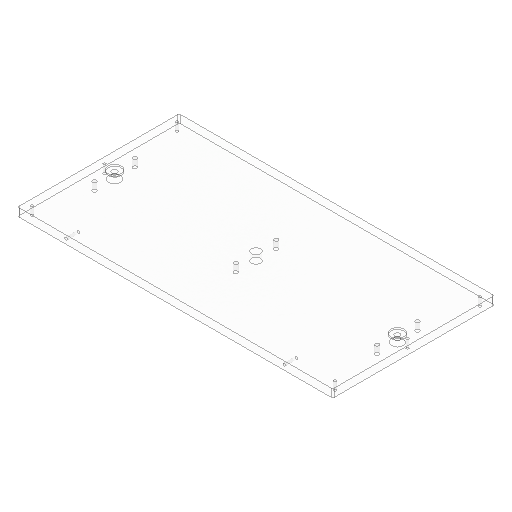
# Autodesk Inventor part: DLT-01-231B
Saved by Autodesk Inventor 2025.2 (Build 292293000, 293)
## iProperties
Company: Delta
Created: 2024-10-16
Part Number: DLT-01-231B
Material: Acrílico TP
Document SubType Name: Modeling
Designer: Willian Pinheiro
Density: 1.19 g/cm^3
Appearance: Transparent - Clear
Project: DLT
Description: Base Pressor B
Mass: 923.478 g
Surface Area: 1693.15 cm^2
Volume: 776.032 cm^3
Acabamento: N/A
Dimensões: 10 x 200 x 390 mm
Total: 1
Author: Willian Pinheiro
Revision Number: 00
Autodesk Inventor part; units mm, degrees
ref_plane "YZ Plane" through (0, 0, 0) normal (1, 0, 0) x (0, 1, 0)
ref_plane "XZ Plane" through (0, 0, 0) normal (0, 1, 0) x (-1, 0, 0)
ref_plane "XY Plane" through (0, 0, 0) normal (0, 0, 1) x (1, 0, 0)
sketch "Sketch1" plane through (0, 0, 0) normal (0, 0, 1) x (1, 0, 0)
  line L0 (0, -252.5291) -> (0, 252.5291) construction
  line L1 (-273, 0) -> (273, 0) construction
  line L2 (-195, 100) -> (195, 100)
  line L3 (195, 100) -> (195, -100)
  line L4 (195, -100) -> (-195, -100)
  line L5 (-195, -100) -> (-195, 100)
  line L6 (-178.1654, -28.1654) -> (-178.1654, 28.1654) construction
  line L7 (-178.1654, 28.1654) -> (178.1654, 28.1654) construction
  line L8 (178.1654, 28.1654) -> (178.1654, -28.1654) construction
  line L9 (178.1654, -28.1654) -> (-178.1654, -28.1654) construction
  circle A0 centre (0, 0) radius 180.3779 construction
  line L10 (-175, 25) -> (-175, -25) construction
  line L11 (-175, -25) -> (175, -25) construction
  line L12 (175, -25) -> (175, 25) construction
  line L13 (175, 25) -> (-175, 25) construction
  circle A1 centre (-175, 0) radius 6 construction
  point P0 (175, 0)
  point P1 (0, 25)
  point P2 (0, -25)
  dimension "d0" = 390
  dimension "d1" = 200
  dimension "d5" = 350
  dimension "d6" = 360.7559
  dimension "d14" = 350
  dimension "d15" = 12
  dimension "d54" = 353.5534
  dimension "d104" = 350
  dimension "d105" = 50
  constraints: 24 end point, 7 parallel, 6 coincident, 3 perpendicular, 3 point on circle, 2 centre point, 2 midpoint, 1 horizontal, 1 point on line, 1 symmetric about line, 5 other
  measures "d0" distance of L2.start L2.end
  measures "d1" distance between parallel lines of L4 L2
  measures "d5" distance between parallel lines of L12 L10
  measures "d6" diameter of A0
  measures "d14" distance of point (175, 0) point (-175, 0)
  measures "d15" diameter of A1
  measures "d54" distance of point (175, 25) point (-175, -25)
  measures "d104" distance of L12.end L10.start
  measures "d105" distance of L10.start L10.end
extrude "Extrusion1" add sketch "Sketch1" along normal blind 10
sketch "Sketch2" plane through (0, 0, 10) normal (0, 0, 1) x (1, 0, 0)
  point P0 (0, 0)
  point P1 (-175, -25)
  point P2 (-175, 25)
  point P3 (175, 25)
  point P4 (175, -25)
  point P5 (-175, 0)
  point P6 (175, 0)
  point P7 (0, 25)
  point P8 (0, -25)
hole "Hole1" at (-175, -25, 10) at (175, 25, 10) at (-175, 25, 10) at (175, -25, 10) at (0, 25, 10) at (0, -25, 10) direction (0, 0, -1) diameter 4.917 end through all thread size "M6x1" class "6H" standard "ISO Metric profile"
hole "Hole2" at (-175, 0, 10) at (175, 0, 10) direction (0, 0, -1) diameter 6.5 end through all counterbore diameter 16.5 counterbore depth 2
sketch "Sketch3" plane through (0, 0, 10) normal (0, 0, 1) x (1, 0, 0)
  line L0 (195, 100) -> (-195, 100) construction
  line L1 (-195, -100) -> (195, -100) construction
  line L2 (-195, 100) -> (-195, -100) construction
  line L3 (-273, 0) -> (273, 0) construction
  line L4 (0, -140) -> (0, 140) construction
  line L5 (195, -100) -> (195, 100) construction
  line L6 (-180, 90) -> (180, 90) construction
  line L7 (180, 90) -> (180, -90) construction
  line L8 (180, -90) -> (-180, -90) construction
  line L9 (-180, -90) -> (-180, 90) construction
  point P0 (0, 0)
  point P1 (-170, 80)
  point P2 (-150, 80)
  point P3 (-150, 80)
  point P4 (-130, 80)
  point P5 (-110, 80)
  point P6 (-90, 80)
  point P7 (-70, 80)
  point P8 (-50, 80)
  point P9 (-30, 80)
  point P10 (-10, 80)
  point P11 (10, 80)
  point P12 (30, 80)
  point P13 (50, 80)
  point P14 (70, 80)
  point P15 (90, 80)
  point P16 (110, 80)
  point P17 (130, 80)
  point P18 (150, 80)
  point P19 (170, 80)
  point P20 (-170, 60)
  point P21 (-150, 60)
  point P22 (-130, 60)
  point P23 (-110, 60)
  point P24 (-90, 60)
  point P25 (-70, 60)
  point P26 (-50, 60)
  point P27 (-30, 60)
  point P28 (-10, 60)
  point P29 (10, 60)
  point P30 (30, 60)
  point P31 (50, 60)
  point P32 (70, 60)
  point P33 (90, 60)
  point P34 (110, 60)
  point P35 (130, 60)
  point P36 (150, 60)
  point P37 (170, 60)
  point P38 (-170, 40)
  point P39 (-150, 40)
  point P40 (-130, 40)
  point P41 (-110, 40)
  point P42 (-90, 40)
  point P43 (-70, 40)
  point P44 (-50, 40)
  point P45 (-30, 40)
  point P46 (-10, 40)
  point P47 (10, 40)
  point P48 (30, 40)
  point P49 (50, 40)
  point P50 (70, 40)
  point P51 (90, 40)
  point P52 (110, 40)
  point P53 (130, 40)
  point P54 (150, 40)
  point P55 (170, 40)
  point P56 (-170, 20)
  point P57 (-150, 20)
  point P58 (-130, 20)
  point P59 (-110, 20)
  point P60 (-90, 20)
  point P61 (-70, 20)
  point P62 (-50, 20)
  point P63 (-30, 20)
  point P64 (-10, 20)
  point P65 (10, 20)
  point P66 (30, 20)
  point P67 (50, 20)
  point P68 (70, 20)
  point P69 (90, 20)
  point P70 (110, 20)
  point P71 (130, 20)
  point P72 (150, 20)
  point P73 (170, 20)
  point P74 (-170, 0)
  point P75 (-150, 0)
  point P76 (-130, 0)
  point P77 (-110, 0)
  point P78 (-90, 0)
  point P79 (-70, 0)
  point P80 (-50, 0)
  point P81 (-30, 0)
  point P82 (-10, 0)
  point P83 (10, 0)
  point P84 (30, 0)
  point P85 (50, 0)
  point P86 (70, 0)
  point P87 (90, 0)
  point P88 (110, 0)
  point P89 (130, 0)
  point P90 (150, 0)
  point P91 (170, 0)
  point P92 (-170, -20)
  point P93 (-150, -20)
  point P94 (-130, -20)
  point P95 (-110, -20)
  point P96 (-90, -20)
  point P97 (-70, -20)
  point P98 (-50, -20)
  point P99 (-30, -20)
  point P100 (-10, -20)
  point P101 (10, -20)
  point P102 (30, -20)
  point P103 (50, -20)
  point P104 (70, -20)
  point P105 (90, -20)
  point P106 (110, -20)
  point P107 (130, -20)
  point P108 (150, -20)
  point P109 (170, -20)
  point P110 (-170, -40)
  point P111 (-150, -40)
  point P112 (-130, -40)
  point P113 (-110, -40)
  point P114 (-90, -40)
  point P115 (-70, -40)
  point P116 (-50, -40)
  point P117 (-30, -40)
  point P118 (-10, -40)
  point P119 (10, -40)
  point P120 (30, -40)
  point P121 (50, -40)
  point P122 (70, -40)
  point P123 (90, -40)
  point P124 (110, -40)
  point P125 (130, -40)
  point P126 (150, -40)
  point P127 (170, -40)
  point P128 (-170, -60)
  point P129 (-150, -60)
  point P130 (-130, -60)
  point P131 (-110, -60)
  point P132 (-90, -60)
  point P133 (-70, -60)
  point P134 (-50, -60)
  point P135 (-30, -60)
  point P136 (-10, -60)
  point P137 (10, -60)
  point P138 (30, -60)
  point P139 (50, -60)
  point P140 (70, -60)
  point P141 (90, -60)
  point P142 (110, -60)
  point P143 (130, -60)
  point P144 (150, -60)
  point P145 (170, -60)
  point P146 (-170, -80)
  point P147 (-150, -80)
  point P148 (-130, -80)
  point P149 (-110, -80)
  point P150 (-90, -80)
  point P151 (-70, -80)
  point P152 (-50, -80)
  point P153 (-30, -80)
  point P154 (-10, -80)
  point P155 (10, -80)
  point P156 (30, -80)
  point P157 (50, -80)
  point P158 (70, -80)
  point P159 (90, -80)
  point P160 (110, -80)
  point P161 (130, -80)
  point P162 (150, -80)
  point P163 (170, -80)
  dimension "d25" = 10
  dimension "d26" = 360
  dimension "d27" = 180
  dimension "d28" = 10
  dimension "d29" = 10
  dimension "d30" = 20
  dimension "d33" = 20
  dimension "d36" = 20
  dimension "d39" = 15
  constraints: 8 end point, 1 horizontal, 1 horizontal alignment, 1 vertical, 163 other
  measures "d25" distance between parallel lines of L0 L6
  measures "d26" distance between parallel lines of L7 L9
  measures "d27" distance between parallel lines of L8 L6
  measures "d28" distance from line of point (-170, 80) L9
  measures "d29" distance from line of point (-170, 80) L6
  measures "d30" distance of point (-150, 80) point (-170, 80)
  measures "d33" distance of point (-170, 80) point (-150, 80)
  measures "d36" distance of point (-170, 80) point (-170, 60)
  measures "d39" distance between parallel lines of L2 L9
hole "Hole3" [suppressed]
hole "Hole4" at (0, 0, 10) direction (0, 0, -1) diameter 11 end through all
sketch "Sketch4" plane through (0, 0, 0) normal (0, 0, -1) x (-1, 0, 0)
  circle A0 centre (175, 0) radius 3.25 construction
  circle A1 centre (-175, 0) radius 3.25 construction
  line L0 (195, -100) -> (-195, -100) construction
  line L1 (187.5, -100) -> (187.5, 100) construction
  line L2 (-195, 100) -> (195, 100) construction
  line L3 (273, 0) -> (-273, 0) construction
  line L4 (0, -140) -> (0, 140) construction
  line L5 (195, 100) -> (195, -100) construction
  point P0 (0, 0)
  point P1 (187.5, -90)
  point P2 (187.5, 90)
  point P3 (187.5, 0)
  point P4 (-187.5, -90)
  point P5 (-187.5, 90)
  point P6 (-187.5, 0)
  dimension "d62" = 180
  dimension "d63" = 7.5
  constraints: 4 point on line, 4 symmetric about line, 2 coincident, 2 end point, 1 midpoint, 1 vertical
  measures "d62" distance of point (187.5, 90) point (187.5, -90)
  measures "d63" distance between parallel lines of L1 L5
hole "Hole5" at (-175, 0, 0) at (175, 0, 0) direction (0, 0, 1) diameter 6.5 end through all countersink diameter 14.5 countersink angle 90 clearance for "Countersunk Flat Head Hex Socket Screw ISO 10642" size "M6" standard "ISO"
hole "Hole6" at (-187.5, -90, 0) at (-187.5, 90, 0) at (-187.5, 0, 0) at (187.5, -90, 0) at (187.5, 0, 0) at (187.5, 90, 0) direction (0, 0, 1) diameter 3.242 end through all thread size "M4x0.7" class "6H" standard "ISO Metric profile"
sketch "Sketch10" plane through (-195, -100, 0) normal (0, -1, 0) x (1, 0, 0)
  line L0 (0, 0) -> (0, 10) construction
  line L1 (0, 6) -> (390, 6) construction
  line L2 (390, 0) -> (390, 10) construction
  line L3 (195, -2) -> (195, 12) construction
  line L4 (0, 10) -> (390, 10) construction
  line L5 (0, 0) -> (390, 0) construction
  point P0 (195, 0)
  point P1 (60, 6)
  point P2 (330, 6)
  dimension "d95" = 270
  dimension "d103" = 6
  constraints: 3 point on line, 2 end point, 1 parallel, 1 symmetric about line
  measures "d95" distance of point (330, 6) point (60, 6)
  measures "d103" distance between parallel lines of L5 L1
hole "Hole10" at (-135, -100, 6) at (135, -100, 6) direction (0, 1, 0) diameter 3.242 depth 15 tip angle 118 thread size "M4x0.7" class "6H" standard "ISO Metric profile"
fillet "Fillet1" radius 2 4 edges at (-195, -100, 5) (195, -100, 5) (-195, 100, 5) (195, 100, 5)
equation "\"d33\" = d30"
equation "\"d36\" = d30"
body "Solid1"
